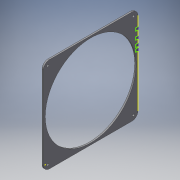
# Autodesk Inventor part: TrayPanelD_180mm
Saved by Autodesk Inventor 2017 (Build 210142000, 142)
## iProperties
Created: 2019-06-22
Part Number: TrayPanelD_180mm
Material: Generic
Document SubType Name: Modeling
Designer: DDeGo
Density: 1 g/cm^3
Appearance: Default
Author: DDeGo
Autodesk Inventor part; units mm, degrees
ref_plane "YZ Plane" through (0, 0, 0) normal (1, 0, 0) x (0, 1, 0)
ref_plane "XZ Plane" through (0, 0, 0) normal (0, 1, 0) x (-1, 0, 0)
ref_plane "XY Plane" through (0, 0, 0) normal (0, 0, 1) x (1, 0, 0)
sketch "Sketch1" plane through (0, 0, 0) normal (1, 0, 0) x (0, 1, 0)
  circle A0 centre (-4, -4) radius 2
  circle A1 centre (78.5, 78.5) radius 85
  circle A2 centre (161, -4) radius 2
  circle A3 centre (-4, 161) radius 2
  circle A4 centre (161, 161) radius 2
  line L0 (157, 170) -> (0, 170)
  arc A5 (0, 170) -> (-13, 157) centre (0, 157) ccw
  line L1 (-13, 157) -> (-13, 0)
  arc A6 (-13, 0) -> (0, -13) centre (0, 0) ccw
  line L2 (0, -13) -> (157, -13)
  arc A7 (157, -13) -> (170, 0) centre (157, 0) ccw
  line L3 (170, 0) -> (170, 157)
  arc A8 (170, 157) -> (157, 170) centre (157, 157) ccw
  line L4 (-4, 161) -> (161, 161) construction
  line L5 (161, 161) -> (161, -4) construction
  line L6 (161, -4) -> (-4, -4) construction
  line L7 (-4, -4) -> (-4, 161) construction
  line L8 (-4, 161) -> (161, -4) construction
  line L9 (-13, 78.5) -> (78.5, 78.5) construction
  line L10 (78.5, 78.5) -> (170, 78.5) construction
  dimension "d10" = 183
  dimension "d11" = 183
  dimension "d12" = 165
  dimension "d13" = 165
  dimension "d15" = 13
  dimension "d16" = 4
  dimension "d17" = 170
  constraints: 22 end point, 9 centre point, 8 point on circle, 8 tangent, 6 equal radius, 3 horizontal, 3 midpoint, 3 perpendicular, 1 coincident, 1 collinear, 1 vertical
  measures "d10" distance between parallel lines of L3 L1
  measures "d11" distance between parallel lines of L0 L2
  measures "d12" distance between parallel lines of L5 L7
  measures "d13" distance of L4.end L5.end
  measures "d15" radius of A5
  measures "d16" diameter of A4
  measures "d17" diameter of A1
extrude "Extrusion1" add sketch "Sketch1" along normal blind 2.75
sketch "Sketch2" plane through (2.75, 0, 0) normal (1, 0, 0) x (0, 0, -1)
  line L0 (0, 170) -> (-157, 170) projected
  line L1 (-146.1, 170) -> (-131.1, 170)
  line L2 (-131.1, 170) -> (-131.1, 166.5)
  line L3 (-131.1, 166.5) -> (-146.1, 166.5)
  line L4 (-146.1, 166.5) -> (-146.1, 170)
  line L5 (-116.1, 170) -> (-101.1, 170)
  line L6 (-101.1, 170) -> (-101.1, 166.5)
  line L7 (-101.1, 166.5) -> (-116.1, 166.5)
  line L8 (-116.1, 166.5) -> (-116.1, 170)
  line L9 (-47.1, 170) -> (-32.1, 170)
  line L10 (-32.1, 170) -> (-32.1, 166.5)
  line L11 (-32.1, 166.5) -> (-47.1, 166.5)
  line L12 (-47.1, 166.5) -> (-47.1, 170)
  line L13 (-2.1, 170) -> (-17.1, 170)
  line L14 (-17.1, 170) -> (-17.1, 166.5)
  line L15 (-17.1, 166.5) -> (-2.1, 166.5)
  line L16 (-2.1, 166.5) -> (-2.1, 170)
  circle A0 centre (-161, 161) radius 2 projected
  point P0 (0, 0)
  dimension "d2" = 15
  dimension "d3" = 30
  dimension "d4" = 69
  dimension "d5" = 30
  dimension "d6" = 3.5
  dimension "d7" = 14.9
  constraints: 32 end point, 8 parallel, 7 point on line, 4 horizontal, 4 perpendicular, 3 collinear
  measures "d2" distance of L2.end L3.end
  measures "d3" distance between parallel lines of L6 L2
  measures "d4" distance between parallel lines of L10 L6
  measures "d5" distance between parallel lines of L16 L10
  measures "d6" distance of L15.end L13.start
  measures "d7" distance from line of L4 A0.centre
extrude "Extrusion2" cut sketch "Sketch2" against normal blind 10 contours L16 L15 L14 L0 | L10 L11 L12 L0 | L6 L7 L8 L0 | L2 L3 L4 L0
sketch "Sketch3" plane through (2.75, 0, 0) normal (1, 0, 0) x (0, 0, -1)
  line L0 (-56, -11) -> (-39.9097, -11)
  line L1 (-39.9097, -11) -> (-39.9097, -8.2)
  line L2 (-39.9097, -8.2) -> (-56, -8.2)
  line L3 (-56, -8.2) -> (-56, -11)
  line L4 (-26, -11) -> (-9.9097, -11)
  line L5 (-9.9097, -11) -> (-9.9097, -8.2)
  line L6 (-9.9097, -8.2) -> (-26, -8.2)
  line L7 (-26, -8.2) -> (-26, -11)
  line L8 (-104.9097, -11) -> (-121, -11)
  line L9 (-121, -11) -> (-121, -8.2)
  line L10 (-121, -8.2) -> (-104.9097, -8.2)
  line L11 (-104.9097, -8.2) -> (-104.9097, -11)
  line L12 (-134.9097, -11) -> (-151, -11)
  line L13 (-151, -11) -> (-151, -8.2)
  line L14 (-151, -8.2) -> (-134.9097, -8.2)
  line L15 (-134.9097, -8.2) -> (-134.9097, -11)
  line L16 (-157, -13) -> (0, -13) projected
  circle A0 centre (-161, -4) radius 2 projected
  point P0 (0, 0)
  dimension "d18" = 2
  dimension "d19" = 30
  dimension "d20" = 65
  dimension "d21" = 30
  dimension "d22" = 2.8
  dimension "d23" = 10
  constraints: 32 end point, 8 parallel, 6 point on line, 4 horizontal, 4 perpendicular, 3 collinear
  measures "d18" distance between parallel lines of L16 L12
  measures "d19" distance between parallel lines of L11 L15
  measures "d20" distance between parallel lines of L1 L11
  measures "d21" distance between parallel lines of L5 L1
  measures "d22" distance of L4.end L5.end
  measures "d23" distance from line of A0.centre L13
extrude "Extrusion3" cut sketch "Sketch3" against normal blind 10 contours L3 L2 L1 L0 | L7 L6 L5 L4 | L8 L9 L10 L11 | L12 L13 L14 L15
body "Solid1"
